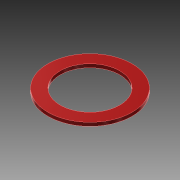
# Autodesk Inventor part: Втулка
Saved by Autodesk Inventor 2022 (Build 260153000, 153)
## iProperties
RuleStatus: InUse
Part Number: Втулка
Checked By: Якушев
Engr Approved By: Малов
Material: По умолчанию1
Document SubType Name: Modeling
Mfg Approved By: Судаков
Designer: Смирнов
Density: 1 g/cm^3
Appearance: Гладкий — красный
AfterMaterialChange0: Материал
BeforeDocSave0: Материал
AfterAnyiPropertyChange0: Материал
Материал: По умолчанию1
Author: Смирнов
Autodesk Inventor part; units mm, degrees
ref_plane "YZ Plane" through (0, 0, 0) normal (1, 0, 0) x (0, 1, 0)
ref_plane "XZ Plane" through (0, 0, 0) normal (0, 1, 0) x (-1, 0, 0)
ref_plane "XY Plane" through (0, 0, 0) normal (0, 0, 1) x (1, 0, 0)
sketch "Эскиз1" plane through (0, 0, 0) normal (0, 0, 1) x (1, 0, 0)
  circle A0 centre (0, 0) radius 4.25
  circle A1 centre (0, 0) radius 6
  dimension "d0" = 8.5
  dimension "d4" = 12
  constraints: 2 centre point, 2 coincident
  measures "d0" diameter of A0
  measures "d4" diameter of A1
extrude "Выдавливание1" add sketch "Эскиз1" along normal mid plane 0.5
